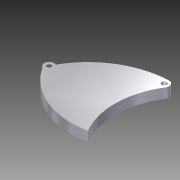
# Autodesk Inventor part: blad
Saved by Autodesk Inventor 2015 (Build 190159000, 159)
## iProperties
Created: 2015-02-05
Part Number: blad
Material: Generic
Document SubType Name: Modeling
Designer: janov_000
Density: 1 g/cm^3
Appearance: Aluminum - Flat
Author: janov_000
Autodesk Inventor part; units mm, degrees
ref_plane "YZ Plane" through (0, 0, 0) normal (1, 0, 0) x (0, 1, 0)
ref_plane "XZ Plane" through (0, 0, 0) normal (0, 1, 0) x (-1, 0, 0)
ref_plane "XY Plane" through (0, 0, 0) normal (0, 0, 1) x (1, 0, 0)
sketch "Sketch1" plane through (0, 0, 0) normal (0, 0, 1) x (1, 0, 0)
  circle A0 centre (0, 0) radius 75 construction
  arc A1 (-78.5195, 32.5529) -> (0, 0) centre (-15.5934, 73.3611) ccw
  line L0 (-15.5934, 73.3611) -> (-78.5195, 32.5529) construction
  line L1 (-15.5934, 73.3611) -> (0, 0) construction
  line L2 (0, 0) -> (64.9519, 37.5) construction
  arc A2 (6.6958, 84.7359) -> (0, 0) centre (64.9519, 37.5) ccw
  line L3 (64.9519, 37.5) -> (6.6958, 84.7359) construction
  line L4 (64.9519, 37.5) -> (0, 0) construction
  line L5 (0, 0) -> (0, 75) construction
  circle A3 centre (0, 0) radius 85 construction
  arc A4 (6.6958, 84.7359) -> (-78.5195, 32.5529) centre (0, 0) ccw
  arc A5 (-74.153, 41.5492) -> (-78.5195, 32.5529) centre (-76.3362, 37.0511) ccw
  line L6 (-76.3362, 37.0511) -> (-78.5195, 32.5529) construction
  line L7 (-76.3362, 37.0511) -> (-74.153, 41.5492) construction
  point P0 (0, 0)
  dimension "d1" = 72
  dimension "d4" = 60
  dimension "d21" = 170
  dimension "d39" = 5
  dimension "d40" = 180
  constraints: 16 end point, 15 point on circle, 5 centre point, 3 coincident, 1 vertical
  measures "d1" angle of L1 L2
  measures "d4" angle of L5 L2
  measures "d21" diameter of A3
  measures "d39" radius of A5
  measures "d40" angle of L7 L6
extrude "Extrusion1" add sketch "Sketch1" along normal blind 10
sketch "Sketch3" plane through (0, 0, 10) normal (0, 0, 1) x (1, 0, 0)
  circle A0 centre (0, 0) radius 80 construction
  circle A1 centre (64.9519, 37.5) radius 75 projected
  circle A2 centre (64.9519, 37.5) radius 80 construction
  point P0 (0, 0)
  point P1 (-2.8573, 79.949)
  dimension "d25" = 160
  dimension "d26" = 160
  constraints: 2 coincident, 6 other
hole "Hole2" at (-2.8573, 79.949, 10) direction (0, 0, -1) diameter 5 end through all
sketch "Sketch4" plane through (0, 0, 10) normal (0, 0, 1) x (1, 0, 0)
  circle A0 centre (-2.8573, 79.949) radius 2.5 projected
  arc A1 (-78.5195, 32.5529) -> (0, 0) centre (-15.5934, 73.3611) ccw projected
  arc A2 (6.6958, 84.7359) -> (1.3808, 77.2959) centre (64.9519, 37.5) ccw
  arc A3 (6.6958, 84.7359) -> (-3.0359, 84.9458) centre (0, 0) ccw
  arc A4 (6.6958, 84.7359) -> (0, 0) centre (64.9519, 37.5) ccw projected
  arc A5 (6.6958, 84.7359) -> (-78.5195, 32.5529) centre (0, 0) ccw projected
  circle A6 centre (-2.8573, 79.949) radius 5
  constraints: 6 centre point, 6 point on circle, 1 coincident, 1 tangent
extrude "Extrusion2" cut sketch "Sketch4" against normal blind 10 contours A3 A2 A6
sketch "Sketch5" plane through (0, 0, 10) normal (0, 0, 1) x (1, 0, 0)
  arc A0 (1.3808, 77.2959) -> (-3.0359, 84.9458) centre (-2.8573, 79.949) ccw projected
  arc A1 (-3.0359, 84.9458) -> (-74.153, 41.5492) centre (0, 0) ccw projected
  arc A2 (-74.153, 41.5492) -> (-78.5195, 32.5529) centre (-76.3362, 37.0511) ccw projected
  arc A3 (-78.5195, 32.5529) -> (0, 0) centre (-15.5934, 73.3611) ccw projected
  arc A4 (1.3808, 77.2959) -> (0, 0) centre (64.9519, 37.5) ccw projected
  circle A5 centre (-2.8573, 79.949) radius 2.5 projected
  point P0 (0, 0)
  constraints: 1 coincident
hole "Hole3" at (-76.3362, 37.0511, 10) direction (0, 0, -1) diameter 4.134 end through all thread size "M5x0.8" class "6H" standard "ANSI Metric M Profile"
sketch "Sketch7" plane through (0, 0, 0) normal (0, 0, -1) x (-1, 0, 0)
  circle A0 centre (76.3362, 37.0511) radius 2.067 projected
  arc A1 (3.0359, 84.9458) -> (-1.3808, 77.2959) centre (2.8573, 79.949) ccw projected
  arc A2 (0, 0) -> (-1.3808, 77.2959) centre (-64.9519, 37.5) ccw projected
  arc A3 (0, 0) -> (78.5195, 32.5529) centre (15.5934, 73.3611) ccw projected
  arc A4 (78.5195, 32.5529) -> (74.153, 41.5492) centre (76.3362, 37.0511) ccw projected
  arc A5 (74.153, 41.5492) -> (3.0359, 84.9458) centre (0, 0) ccw projected
  circle A6 centre (2.8573, 79.949) radius 2.5 projected
  arc A7 (71.5064, 35.8724) -> (12.5647, 79.0071) centre (0, 0) ccw
  arc A8 (14.8454, 3.3651) -> (70.9945, 30.5742) centre (15.5934, 73.3611) ccw
  arc A9 (10.2017, 10.0786) -> (7.2658, 71.9181) centre (-64.9519, 37.5) ccw
  arc A10 (10.2017, 10.0786) -> (14.8454, 3.3651) centre (14.8988, 8.3648) ccw
  arc A11 (12.5647, 79.0071) -> (7.2658, 71.9181) centre (11.7794, 74.0692) ccw
  arc A12 (70.9945, 30.5742) -> (71.5064, 35.8724) centre (67.0373, 33.6304) ccw
  point P0 (0, 0)
  dimension "d51" = 5
  dimension "d55" = 5
  constraints: 12 point on circle, 6 centre point, 6 tangent, 2 equal radius, 2 other
  measures "d51" radial gap between concentric circles of A2 A9
  measures "d55" radius of A10
extrude "Extrusion4" cut sketch "Sketch7" against normal blind 2 contours A12 A8 A10 A9 A11 A7
body "Solid1"
